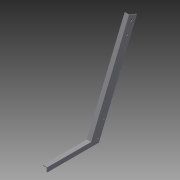
# Autodesk Inventor part: CatapultArmZ-Right
Saved by Autodesk Inventor 2013 (Build 170138000, 138)
## iProperties
Created: 2014-01-20
Part Number: CatapultArmZ-Right
Material: Generic
Document SubType Name: Modeling
Designer: RobertB
Density: 1 g/cm^3
Author: RobertB
Autodesk Inventor part; units mm, degrees
ref_plane "YZ Plane" through (0, 0, 0) normal (1, 0, 0) x (0, 1, 0)
ref_plane "XZ Plane" through (0, 0, 0) normal (0, 1, 0) x (-1, 0, 0)
ref_plane "XY Plane" through (0, 0, 0) normal (0, 0, 1) x (1, 0, 0)
sketch "Sketch1" plane through (0, 0, 0) normal (1, 0, 0) x (0, 1, 0)
  line L0 (0, 0) -> (0, 254)
  line L1 (0, 0) -> (254, 0) construction
  line L2 (0, 0) -> (527.9972, -218.7036)
  line L3 (0, 0) -> (571.5, 0) construction
  line L4 (0, 254) -> (-25.4, 254)
  line L5 (0, 254) -> (25.4, 254) construction
  line L6 (527.9972, -218.7036) -> (508.5568, -265.6367)
  line L7 (527.9972, -218.7036) -> (578.7972, -218.7036) construction
  line L8 (508.5568, -265.6367) -> (-19.4403, -46.9331)
  line L9 (-19.4403, -46.9331) -> (-6.7403, -46.9331) construction
  line L10 (-25.4, 254) -> (-25.4, -44.4645)
  line L11 (-25.4, 254) -> (273.0645, 254) construction
  line L12 (-25.4, -44.4645) -> (-19.4403, -46.9331)
  line L13 (518.277, -242.1701) -> (543.677, -242.1701) construction
  circle A0 centre (494.8105, -232.45) radius 6.35
  circle A1 centre (436.1441, -208.1496) radius 6.35
  line L14 (-19.4403, -46.9331) -> (-14.5802, -35.1998)
  line L15 (126.219, -93.5208) -> (121.3589, -105.254)
  line L16 (-14.5802, -35.1998) -> (-1.8802, -35.1998) construction
  line L17 (-2.847, -40.0599) -> (86.053, -40.0599) construction
  circle A2 centre (79.2859, -74.0804) radius 3.175
  circle A3 centre (-2.847, -40.0599) radius 3.175
  dimension "d0" = 254
  dimension "d1" = 90
  dimension "d2" = 571.5
  dimension "d3" = 22.5
  dimension "d4" = 25.4
  dimension "d5" = 180
  dimension "d6" = 50.8
  dimension "d7" = 112.5
  dimension "d8" = 571.5
  dimension "d9" = 90
  dimension "d12" = 90
  dimension "d17" = 12.7
  dimension "d18" = 12.7
  dimension "d19" = 12.7
  dimension "d20" = 152.4
  dimension "d22" = 12.7
  dimension "d26" = 6.35
  dimension "d27" = 6.35
  constraints: 36 end point, 9 horizontal, 5 equal length, 4 centre point, 3 perpendicular, 1 coincident, 1 midpoint, 1 parallel, 1 point on line, 1 vertical
  measures "d0" distance of L0.start L0.end
  measures "d1" angle of L1 L0
  measures "d2" distance of L0.start L2.end
  measures "d3" angle of L2 L3
  measures "d4" distance of L0.end L4.end
  measures "d5" angle of L4 L5
  measures "d6" distance of L2.end L6.end
  measures "d7" angle of L6 L7
  measures "d8" distance of L6.end L8.end
  measures "d9" angle of L6 L8
  measures "d12" angle of L10 L11
  measures "d17" diameter of A0
  measures "d18" diameter of A1
  measures "d19" distance of L8.end L14.end
  measures "d20" distance of L14.end L15.start
  measures "d22" distance of L14.end L17.start
  measures "d26" diameter of A2
  measures "d27" diameter of A3
extrude "Extrusion1" add sketch "Sketch1" along normal blind 3.175
sketch "Sketch2" plane through (3.175, 0, 0) normal (1, 0, 0) x (0, 0, -1)
  line L0 (0, 0) -> (-254, 0) projected
  line L1 (265.6367, 508.5568) -> (218.7036, 527.9972) projected
  line L2 (218.7036, 527.9972) -> (0, 0) projected
  line L3 (218.7036, 527.9972) -> (221.6369, 526.7821)
  line L4 (218.7036, 527.9972) -> (221.8786, 527.9972) construction
  line L5 (-254, 0) -> (-254, -3.175)
  line L6 (-254, 0) -> (-250.825, 0) construction
  line L7 (-254, -3.175) -> (2.1215, -3.175)
  line L8 (2.1215, -3.175) -> (221.6369, 526.7821)
  dimension "d30" = 3.175
  dimension "d31" = 22.5
  dimension "d33" = 3.175
  dimension "d34" = 90
  dimension "d35" = 90
  constraints: 12 end point, 2 equal length, 2 horizontal, 1 collinear, 1 perpendicular
  measures "d30" distance of L1.end L3.end
  measures "d31" angle of L3 L4
  measures "d33" distance of L0.end L5.end
  measures "d34" angle of L5 L6
  measures "d35" angle of L7 L5
extrude "Extrusion2" add sketch "Sketch2" against normal blind 25.4
body "Solid1"
